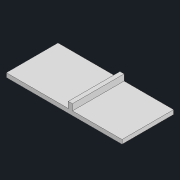
# Autodesk Inventor part: Part2
Saved by Autodesk Inventor 2022 (Build 260153000, 153)
## iProperties
Created: 2021-11-19
Part Number: Part2
Material: 一般
Document SubType Name: Modeling
Designer: Yuta Kage
Density: 1 g/cm^3
Appearance: 既定
Author: Yuta Kage
Autodesk Inventor part; units mm, degrees
ref_plane "YZ Plane" through (0, 0, 0) normal (1, 0, 0) x (0, 1, 0)
ref_plane "XZ Plane" through (0, 0, 0) normal (0, 1, 0) x (-1, 0, 0)
ref_plane "XY Plane" through (0, 0, 0) normal (0, 0, 1) x (1, 0, 0)
sketch "スケッチ1" plane through (0, 0, 0) normal (0, 1, 0) x (-1, 0, 0)
  line L0 (56, 25) -> (-56, 25)
  line L1 (-56, 25) -> (-56, -25)
  line L2 (-56, -25) -> (56, -25)
  line L3 (56, -25) -> (56, 25)
  line L4 (56, 25) -> (-56, -25) construction
  line L5 (-56, 25) -> (56, -25) construction
  point P0 (0, 0)
  dimension "d0" = 112
  dimension "d1" = 50
  constraints: 12 end point, 2 midpoint, 2 parallel, 1 horizontal, 1 perpendicular
  measures "d0" distance of L1.end L2.end
  measures "d1" distance of L0.end L1.end
extrude "押し出し1" add sketch "スケッチ1" along normal blind 10
sketch "スケッチ2" plane through (0, 10, 0) normal (0, 1, 0) x (1, 0, 0)
  line L0 (56, 25) -> (-56, 25) projected
  line L1 (-56, -25) -> (56, -25) projected
  line L2 (-56, 25) -> (4, 25)
  line L3 (4, 25) -> (4, -25)
  line L4 (4, -25) -> (-56, -25)
  line L5 (-56, -25) -> (-56, 25)
  line L6 (56, -25) -> (56, 25) projected
  line L7 (56, 25) -> (8, 25)
  line L8 (8, 25) -> (8, -25)
  line L9 (8, -25) -> (56, -25)
  line L10 (56, -25) -> (56, 25)
  point P0 (0, 0)
  point P1 (4, 25)
  point P2 (8, 25)
  point P3 (8, -25)
  dimension "d4" = 60
  dimension "d5" = 48
  constraints: 16 end point, 4 parallel, 2 horizontal, 2 perpendicular, 2 point on line
  measures "d4" distance between parallel lines of L5 L3
  measures "d5" distance between parallel lines of L6 L8
extrude "押し出し2" cut sketch "スケッチ2" against normal blind 6 contours L6 L1 L8 L0 | L3 L1 L5 L0
